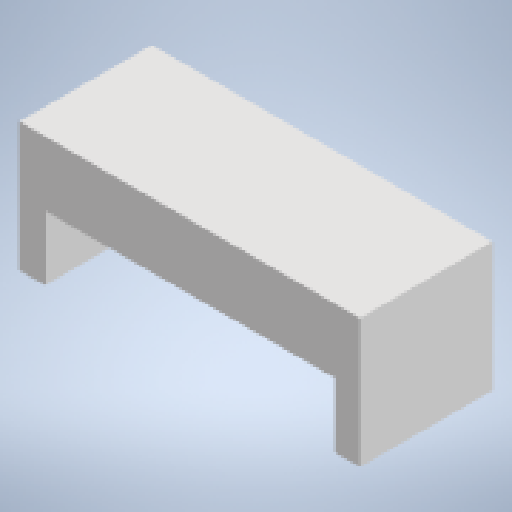
# Autodesk Inventor part: sofa
Saved by Autodesk Inventor 2024 (Build 280153000, 153)
## iProperties
Created: 2023-11-25
Part Number: sofa
Material: Genérico
Document SubType Name: Modeling
Designer: sergi
Density: 1 g/cm^3
Appearance: Valor por defecto
Author: sergi
Autodesk Inventor part; units mm, degrees
ref_plane "YZ Plane" through (0, 0, 0) normal (1, 0, 0) x (0, 1, 0)
ref_plane "XZ Plane" through (0, 0, 0) normal (0, 1, 0) x (-1, 0, 0)
ref_plane "XY Plane" through (0, 0, 0) normal (0, 0, 1) x (1, 0, 0)
sketch "Boceto1" plane through (0, 0, 0) normal (0, 1, 0) x (-1, 0, 0)
  line L0 (0, 0) -> (-1850, 0)
  line L1 (-1850, 0) -> (-1850, -720)
  line L2 (-1850, -720) -> (0, -720)
  line L3 (0, -720) -> (0, 0)
  dimension "d0" = 1850
  dimension "d1" = 720
  constraints: 8 end point, 2 parallel, 1 horizontal, 1 perpendicular
  measures "d0" distance of L2.end L1.end
  measures "d1" distance of L1.end L0.end
extrude "Extrusión1" add sketch "Boceto1" along normal blind 700
sketch "Boceto2" plane through (0, 0, 0) normal (0, -1, 0) x (1, 0, 0)
  line L0 (1850, 0) -> (1850, -720) projected
  line L1 (0, 0) -> (1850, 0) projected
  line L2 (0, -720) -> (0, 0) projected
  line L3 (1850, -720) -> (0, -720) projected
  line L4 (140, -580) -> (140, -140)
  line L5 (1710, -140) -> (1710, -580)
  line L6 (1710, -580) -> (140, -580)
  line L7 (1710, -140) -> (1710, 0)
  line L8 (140, -140) -> (140, 0)
  dimension "d4" = 140
  constraints: 10 end point, 2 point on line, 1 parallel, 1 perpendicular, 1 other
  measures "d4" distance between parallel lines of L3 L6
extrude "Extrusión2" cut sketch "Boceto2" against normal blind 350 contours L7 L5 L6 L4 L8 L1
